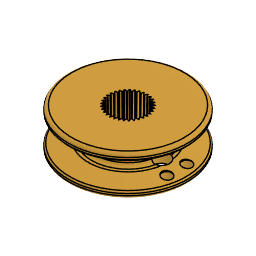
Spool_v5 (Autodesk Fusion 360 design; units mm, degrees)
Autodesk Fusion 360 part; units mm, degrees
note: some values were not read from the file. Set by a fixed rule: which sketch regions a step uses.
sketch "Sketch1" plane through (0, 0, 0) normal (0, 0, 1) x (1, 0, 0)
  line L0 (-0.0246, -2.4999) -> (0.1607, -2.8207)
  line L1 (0.1607, -2.8207) -> (0.3083, -2.4809)
  arc A0 (0.3083, -2.4809) -> (0.449, -2.4594) centre (0, 0) ccw
  line L2 (0.449, -2.4594) -> (0.6916, -2.7393)
  line L3 (0.6916, -2.7393) -> (0.7722, -2.3777)
  arc A1 (0.7722, -2.3777) -> (0.9063, -2.3299) centre (0, 0) ccw
  line L4 (0.9063, -2.3299) -> (1.1975, -2.5589)
  line L5 (1.1975, -2.5589) -> (1.2083, -2.1886)
  arc A2 (1.2083, -2.1886) -> (1.3309, -2.1163) centre (0, 0) ccw
  line L6 (1.3309, -2.1163) -> (1.6601, -2.286)
  line L7 (1.6601, -2.286) -> (1.6006, -1.9204)
  arc A3 (1.6006, -1.9204) -> (1.7073, -1.8262) centre (0, 0) ccw
  line L8 (1.7073, -1.8262) -> (2.0628, -1.9306)
  line L9 (2.0628, -1.9306) -> (1.9351, -1.5828)
  arc A4 (1.9351, -1.5828) -> (2.0221, -1.4701) centre (0, 0) ccw
  line L10 (2.0221, -1.4701) -> (2.3909, -1.5053)
  line L11 (2.3909, -1.5053) -> (2.1997, -1.188)
  arc A5 (2.1997, -1.188) -> (2.2638, -1.0608) centre (0, 0) ccw
  line L12 (2.2638, -1.0608) -> (2.6325, -1.0256)
  line L13 (2.6325, -1.0256) -> (2.3848, -0.7502)
  arc A6 (2.3848, -0.7502) -> (2.4236, -0.6133) centre (0, 0) ccw
  line L14 (2.4236, -0.6133) -> (2.7791, -0.5089)
  line L15 (2.7791, -0.5089) -> (2.4837, -0.2853)
  arc A7 (2.4837, -0.2853) -> (2.4959, -0.1435) centre (0, 0) ccw
  line L16 (2.4959, -0.1435) -> (2.8251, 0.0263)
  line L17 (2.8251, 0.0263) -> (2.4928, 0.1899)
  arc A8 (2.4928, 0.1899) -> (2.4779, 0.3314) centre (0, 0) ccw
  line L18 (2.4779, 0.3314) -> (2.7691, 0.5605)
  line L19 (2.7691, 0.5605) -> (2.4118, 0.6582)
  arc A9 (2.4118, 0.6582) -> (2.3704, 0.7944) centre (0, 0) ccw
  line L20 (2.3704, 0.7944) -> (2.613, 1.0744)
  line L21 (2.613, 1.0744) -> (2.2436, 1.1028)
  arc A10 (2.2436, 1.1028) -> (2.1772, 1.2287) centre (0, 0) ccw
  line L22 (2.1772, 1.2287) -> (2.3625, 1.5495)
  line L23 (2.3625, 1.5495) -> (1.9944, 1.5074)
  arc A11 (1.9944, 1.5074) -> (1.9054, 1.6185) centre (0, 0) ccw
  line L24 (1.9054, 1.6185) -> (2.0265, 1.9686)
  line L25 (2.0265, 1.9686) -> (1.6731, 1.8576)
  arc A12 (1.6731, 1.8576) -> (1.5646, 1.9498) centre (0, 0) ccw
  line L26 (1.5646, 1.9498) -> (1.6173, 2.3165)
  line L27 (1.6173, 2.3165) -> (1.2913, 2.1407)
  arc A13 (1.2913, 2.1407) -> (1.1674, 2.2107) centre (0, 0) ccw
  line L28 (1.1674, 2.2107) -> (1.1497, 2.5807)
  line L29 (1.1497, 2.5807) -> (0.8628, 2.3464)
  arc A14 (0.8628, 2.3464) -> (0.7279, 2.3917) centre (0, 0) ccw
  line L30 (0.7279, 2.3917) -> (0.6405, 2.7517)
  line L31 (0.6405, 2.7517) -> (0.4032, 2.4673)
  arc A15 (0.4032, 2.4673) -> (0.2621, 2.4862) centre (0, 0) ccw
  line L32 (0.2621, 2.4862) -> (0.1082, 2.8232)
  line L33 (0.1082, 2.8232) -> (-0.0711, 2.499)
  arc A16 (-0.0711, 2.499) -> (-0.2132, 2.4909) centre (0, 0) ccw
  line L34 (-0.2132, 2.4909) -> (-0.4281, 2.7926)
  line L35 (-0.4281, 2.7926) -> (-0.5427, 2.4404)
  arc A17 (-0.5427, 2.4404) -> (-0.6807, 2.4055) centre (0, 0) ccw
  line L36 (-0.6807, 2.4055) -> (-0.9488, 2.6612)
  line L37 (-0.9488, 2.6612) -> (-0.9948, 2.2936)
  arc A18 (-0.9948, 2.2936) -> (-1.1237, 2.2332) centre (0, 0) ccw
  line L38 (-1.1237, 2.2332) -> (-1.4353, 2.4335)
  line L39 (-1.4353, 2.4335) -> (-1.4108, 2.0639)
  arc A19 (-1.4108, 2.0639) -> (-1.526, 1.9802) centre (0, 0) ccw
  line L40 (-1.526, 1.9802) -> (-1.8699, 2.1179)
  line L41 (-1.8699, 2.1179) -> (-1.7759, 1.7596)
  arc A20 (-1.7759, 1.7596) -> (-1.8732, 1.6556) centre (0, 0) ccw
  line L42 (-1.8732, 1.6556) -> (-2.2369, 1.7257)
  line L43 (-2.2369, 1.7257) -> (-2.0768, 1.3917)
  arc A21 (-2.0768, 1.3917) -> (-2.1527, 1.2712) centre (0, 0) ccw
  line L44 (-2.1527, 1.2712) -> (-2.5231, 1.2712)
  line L45 (-2.5231, 1.2712) -> (-2.3027, 0.9735)
  arc A22 (-2.3027, 0.9735) -> (-2.3543, 0.8409) centre (0, 0) ccw
  line L46 (-2.3543, 0.8409) -> (-2.7181, 0.7707)
  line L47 (-2.7181, 0.7707) -> (-2.4453, 0.5201)
  arc A23 (-2.4453, 0.5201) -> (-2.4709, 0.3801) centre (0, 0) ccw
  line L48 (-2.4709, 0.3801) -> (-2.8148, 0.2424)
  line L49 (-2.8148, 0.2424) -> (-2.4995, 0.0479)
  arc A24 (-2.4995, 0.0479) -> (-2.4982, -0.0944) centre (0, 0) ccw
  line L50 (-2.4982, -0.0944) -> (-2.8098, -0.2947)
  line L51 (-2.8098, -0.2947) -> (-2.4634, -0.426)
  arc A25 (-2.4634, -0.426) -> (-2.4352, -0.5655) centre (0, 0) ccw
  line L52 (-2.4352, -0.5655) -> (-2.7033, -0.8211)
  line L53 (-2.7033, -0.8211) -> (-2.3383, -0.8845)
  arc A26 (-2.3383, -0.8845) -> (-2.2842, -1.0161) centre (0, 0) ccw
  line L54 (-2.2842, -1.0161) -> (-2.499, -1.3179)
  line L55 (-2.499, -1.3179) -> (-2.1287, -1.311)
  arc A27 (-2.1287, -1.311) -> (-2.0506, -1.4301) centre (0, 0) ccw
  line L56 (-2.0506, -1.4301) -> (-2.2045, -1.767)
  line L57 (-2.2045, -1.767) -> (-1.8421, -1.6902)
  arc A28 (-1.8421, -1.6902) -> (-1.7429, -1.7923) centre (0, 0) ccw
  line L58 (-1.7429, -1.7923) -> (-1.8302, -2.1523)
  line L59 (-1.8302, -2.1523) -> (-1.4889, -2.0083)
  arc A29 (-1.4889, -2.0083) -> (-1.3722, -2.0897) centre (0, 0) ccw
  line L60 (-1.3722, -2.0897) -> (-1.3898, -2.4598)
  line L61 (-1.3898, -2.4598) -> (-1.0819, -2.2538)
  arc A30 (-1.0819, -2.2538) -> (-0.9519, -2.3117) centre (0, 0) ccw
  line L62 (-0.9519, -2.3117) -> (-0.8992, -2.6783)
  line L63 (-0.8992, -2.6783) -> (-0.6359, -2.4178)
  arc A31 (-0.6359, -2.4178) -> (-0.4972, -2.4501) centre (0, 0) ccw
  line L64 (-0.4972, -2.4501) -> (-0.3761, -2.8001)
  line L65 (-0.3761, -2.8001) -> (-0.1668, -2.4944)
  arc A32 (-0.1668, -2.4944) -> (-0.0246, -2.4999) centre (0, 0) ccw
  circle A33 centre (0, 0) radius 9
  circle A34 centre (0, 0) radius 5
  circle A35 centre (5, 0) radius 1.25
  circle A36 centre (0, 0) radius 1.7
  line L66 (7.3721, -1.5) -> (7.3721, 1.5)
  circle A37 centre (7.3721, -1.5) radius 0.75
  circle A38 centre (7.3721, 1.5) radius 0.75
  line L67 (7.3721, -1.5) -> (7.3721, -2.25)
  arc A39 (1.6851, 1.9138) -> (1.6182, 1.9708) centre (0, 0) ccw
  line L68 (1.6182, 1.9708) -> (1.6809, 2.4076)
  line L69 (1.6809, 2.4076) -> (1.2925, 2.1982)
  arc A40 (1.2925, 2.1982) -> (1.2159, 2.2414) centre (0, 0) ccw
  line L70 (1.2159, 2.2414) -> (1.1949, 2.6822)
  line L71 (1.1949, 2.6822) -> (0.8531, 2.4031)
  arc A41 (0.8531, 2.4031) -> (0.7698, 2.431) centre (0, 0) ccw
  line L72 (0.7698, 2.431) -> (0.6657, 2.8599)
  line L73 (0.6657, 2.8599) -> (0.3829, 2.5211)
  arc A42 (0.3829, 2.5211) -> (0.2958, 2.5328) centre (0, 0) ccw
  line L74 (0.2958, 2.5328) -> (0.1124, 2.9342)
  line L75 (0.1124, 2.9342) -> (-0.1011, 2.548)
  arc A43 (-0.1011, 2.548) -> (-0.1889, 2.543) centre (0, 0) ccw
  line L76 (-0.1889, 2.543) -> (-0.4449, 2.9025)
  line L77 (-0.4449, 2.9025) -> (-0.5815, 2.4828)
  arc A44 (-0.5815, 2.4828) -> (-0.6667, 2.4613) centre (0, 0) ccw
  line L78 (-0.6667, 2.4613) -> (-0.9862, 2.7658)
  line L79 (-0.9862, 2.7658) -> (-1.0409, 2.3279)
  arc A45 (-1.0409, 2.3279) -> (-1.1205, 2.2906) centre (0, 0) ccw
  line L80 (-1.1205, 2.2906) -> (-1.4918, 2.5292)
  line L81 (-1.4918, 2.5292) -> (-1.4626, 2.0888)
  arc A46 (-1.4626, 2.0888) -> (-1.5337, 2.0372) centre (0, 0) ccw
  line L82 (-1.5337, 2.0372) -> (-1.9435, 2.2012)
  line L83 (-1.9435, 2.2012) -> (-1.8315, 1.7743)
  arc A47 (-1.8315, 1.7743) -> (-1.8916, 1.7101) centre (0, 0) ccw
  line L84 (-1.8916, 1.7101) -> (-2.3249, 1.7936)
  line L85 (-2.3249, 1.7936) -> (-2.1342, 1.3956)
  arc A48 (-2.1342, 1.3956) -> (-2.181, 1.3212) centre (0, 0) ccw
  line L86 (-2.181, 1.3212) -> (-2.6223, 1.3212)
  line L87 (-2.6223, 1.3212) -> (-2.3597, 0.9665)
  arc A49 (-2.3597, 0.9665) -> (-2.3917, 0.8846) centre (0, 0) ccw
  line L88 (-2.3917, 0.8846) -> (-2.825, 0.801)
  line L89 (-2.825, 0.801) -> (-2.5, 0.5025)
  arc A50 (-2.5, 0.5025) -> (-2.5158, 0.416) centre (0, 0) ccw
  line L90 (-2.5158, 0.416) -> (-2.9255, 0.2519)
  line L91 (-2.9255, 0.2519) -> (-2.5499, 0.0203)
  arc A51 (-2.5499, 0.0203) -> (-2.5491, -0.0677) centre (0, 0) ccw
  line L92 (-2.5491, -0.0677) -> (-2.9204, -0.3063)
  line L93 (-2.9204, -0.3063) -> (-2.5077, -0.4627)
  arc A52 (-2.5077, -0.4627) -> (-2.4902, -0.5489) centre (0, 0) ccw
  line L94 (-2.4902, -0.5489) -> (-2.8096, -0.8534)
  line L95 (-2.8096, -0.8534) -> (-2.3748, -0.9289)
  arc A53 (-2.3748, -0.9289) -> (-2.3414, -1.0102) centre (0, 0) ccw
  line L96 (-2.3414, -1.0102) -> (-2.5973, -1.3697)
  line L97 (-2.5973, -1.3697) -> (-2.1561, -1.3616)
  arc A54 (-2.1561, -1.3616) -> (-2.1079, -1.4351) centre (0, 0) ccw
  line L98 (-2.1079, -1.4351) -> (-2.2912, -1.8365)
  line L99 (-2.2912, -1.8365) -> (-1.8594, -1.745)
  arc A55 (-1.8594, -1.745) -> (-1.7982, -1.8081) centre (0, 0) ccw
  line L100 (-1.7982, -1.8081) -> (-1.9022, -2.2369)
  line L101 (-1.9022, -2.2369) -> (-1.4956, -2.0654)
  arc A56 (-1.4956, -2.0654) -> (-1.4235, -2.1157) centre (0, 0) ccw
  line L102 (-1.4235, -2.1157) -> (-1.4445, -2.5565)
  line L103 (-1.4445, -2.5565) -> (-1.0777, -2.3111)
  arc A57 (-1.0777, -2.3111) -> (-0.9974, -2.3469) centre (0, 0) ccw
  line L104 (-0.9974, -2.3469) -> (-0.9345, -2.7837)
  line L105 (-0.9345, -2.7837) -> (-0.6208, -2.4733)
  arc A58 (-0.6208, -2.4733) -> (-0.5352, -2.4932) centre (0, 0) ccw
  line L106 (-0.5352, -2.4932) -> (-0.3908, -2.9102)
  line L107 (-0.3908, -2.9102) -> (-0.1416, -2.5461)
  arc A59 (-0.1416, -2.5461) -> (-0.0537, -2.5494) centre (0, 0) ccw
  line L108 (-0.0537, -2.5494) -> (0.167, -2.9316)
  line L109 (0.167, -2.9316) -> (0.3428, -2.5268)
  arc A60 (0.3428, -2.5268) -> (0.4298, -2.5135) centre (0, 0) ccw
  line L110 (0.4298, -2.5135) -> (0.7188, -2.847)
  line L111 (0.7188, -2.847) -> (0.8149, -2.4163)
  arc A61 (0.8149, -2.4163) -> (0.8977, -2.3868) centre (0, 0) ccw
  line L112 (0.8977, -2.3868) -> (1.2446, -2.6596)
  line L113 (1.2446, -2.6596) -> (1.2574, -2.2184)
  arc A62 (1.2574, -2.2184) -> (1.3332, -2.1738) centre (0, 0) ccw
  line L114 (1.3332, -2.1738) -> (1.7254, -2.376)
  line L115 (1.7254, -2.376) -> (1.6545, -1.9404)
  arc A63 (1.6545, -1.9404) -> (1.7204, -1.8822) centre (0, 0) ccw
  line L116 (1.7204, -1.8822) -> (2.1439, -2.0065)
  line L117 (2.1439, -2.0065) -> (1.9919, -1.5922)
  arc A64 (1.9919, -1.5922) -> (2.0456, -1.5226) centre (0, 0) ccw
  line L118 (2.0456, -1.5226) -> (2.4849, -1.5645)
  line L119 (2.4849, -1.5645) -> (2.2572, -1.1864)
  arc A65 (2.2572, -1.1864) -> (2.2967, -1.1079) centre (0, 0) ccw
  line L120 (2.2967, -1.1079) -> (2.7361, -1.0659)
  line L121 (2.7361, -1.0659) -> (2.4409, -0.7378)
  arc A66 (2.4409, -0.7378) -> (2.4649, -0.6532) centre (0, 0) ccw
  line L122 (2.4649, -0.6532) -> (2.8883, -0.5289)
  line L123 (2.8883, -0.5289) -> (2.5364, -0.2625)
  arc A67 (2.5364, -0.2625) -> (2.544, -0.1749) centre (0, 0) ccw
  line L124 (2.544, -0.1749) -> (2.9362, 0.0273)
  line L125 (2.9362, 0.0273) -> (2.5403, 0.2222)
  arc A68 (2.5403, 0.2222) -> (2.5311, 0.3097) centre (0, 0) ccw
  line L126 (2.5311, 0.3097) -> (2.878, 0.5825)
  line L127 (2.878, 0.5825) -> (2.4523, 0.699)
  arc A69 (2.4523, 0.699) -> (2.4268, 0.7831) centre (0, 0) ccw
  line L128 (2.4268, 0.7831) -> (2.7158, 1.1166)
  line L129 (2.7158, 1.1166) -> (2.2757, 1.1504)
  arc A70 (2.2757, 1.1504) -> (2.2347, 1.2282) centre (0, 0) ccw
  line L130 (2.2347, 1.2282) -> (2.4554, 1.6104)
  line L131 (2.4554, 1.6104) -> (2.0169, 1.5603)
  arc A71 (2.0169, 1.5603) -> (1.9619, 1.6289) centre (0, 0) ccw
  line L132 (1.9619, 1.6289) -> (2.1062, 2.046)
  line L133 (2.1062, 2.046) -> (1.6851, 1.9138)
  point P0 (7.3721, 0)
  dimension "d1" = 0.05
  dimension "d2" = 18
  dimension "d5" = 10
  dimension "d10" = 2.5
  dimension "d19" = 3.4
  dimension "d24" = 3
  dimension "d25" = 1.5
  dimension "d26" = 1.5
  constraint concentric A0 A33
  constraint concentric A0 A34
  constraint coincident A34 A35.centre
  constraint concentric A33 A36
  constraint midpoint L66 P0
  constraint vertical L66
  constraint coincident L66.start A37.centre
  constraint coincident L66.end A38.centre
  constraint coincident A37 L67.end
  constraint parallel L66 L67
  measures "d2" diameter of A33
  measures "d5" diameter of A34
  measures "d10" diameter of A35
  measures "d19" diameter of A36
  measures "d24" distance of L66.start L66.end
  measures "d25" diameter of A37
  measures "d26" diameter of A38
extrude "Extrude1" add sketch "Sketch1" along normal blind 6 contours A33 | A34 A35 | A34 A35 | A34 A35 | L66 A37 L67 | L66 A37 L67 | A38
extrude "Extrude2" cut sketch "Sketch1" along normal blind 3 from surface at 1.5 contours A33 | A34 A35 | L66 A37 L67 | L66 A37 L67 | A38 picked at (5.374, -0.3105)
extrude "Extrude3" cut sketch "Sketch1" along normal blind 4.5 contours L0 L1 A0 L2 L3 A1 L4 L5 A2 L6 L7 A3 L8 L9 A4 L10 L11 A5 L12 L13 A6 L14 L15 A7 L16 L17 A8 L18 L19 A9 L20 L21 A10 L22 L23 A11 L24 L25 A12 L26 L27 A13 L28 L29 A14 L30 L31 A15 L32 L33 A16 L34 L35 A17 L36 L37 A18 L38 L39 A19 L40 L41 A20 L42 L43 A21 L44 L45 A22 L46 L47 A23 L48 L49 A24 L50 L51 A25 L52 L53 A26 L54 L55 A27 L56 L57 A28 L58 L59 A29 L60 L61 A30 L62 L63 A31 L64 L65 A32 | A34 A35 | A34 A35 | A36 | L66 A37 L67 | L66 A37 L67 | A38 | A39 L68 L69 A40 L70 L71 A41 L72 L73 A42 L74 L75 A43 L76 L77 A44 L78 L79 A45 L80 L81 A46 L82 L83 A47 L84 L85 A48 L86 L87 A49 L88 L89 A50 L90 L91 A51 L92 L93 A52 L94 L95 A53 L96 L97 A54 L98 L99 A55 L100 L101 A56 L102 L103 A57 L104 L105 A58 L106 L107 A59 L108 L109 A60 L110 L111 A61 L112 L113 A62 L114 L115 A63 L116 L117 A64 L118 L119 A65 L120 L121 A66 L122 L123 A67 L124 L125 A68 L126 L127 A69 L128 L129 A70 L130 L131 A71 L132 L133 picked at (4.5948, -0.2579) picked at (5.374, -0.3105)
fillet "Fillet2" radius 0.5 2 edges at (-8.3909, -3.2545, 0) (-8.3909, -3.2545, 6)
chamfer "Chamfer1" distance 0.5 distance2 3 2 edges at (-8.3909, 3.2545, 1.5) (-8.3909, -3.2545, 4.5) measured on face at (8.9553, -0.8961, 0.8333) measured on face at (8.9553, -0.8961, 4.8333) tangent chain off
fillet "Fillet4" radius 0.5 2 edges at (-5, 0, 1.5) (-5, 0, 4.5)
extrude "Extrude4" add sketch "Sketch1" along normal blind 2 contours L0 L1 A0 L2 L3 A1 L4 L5 A2 L6 L7 A3 L8 L9 A4 L10 L11 A5 L12 L13 A6 L14 L15 A7 L16 L17 A8 L18 L19 A9 L20 L21 A10 L22 L23 A11 L24 L25 A12 L26 L27 A13 L28 L29 A14 L30 L31 A15 L32 L33 A16 L34 L35 A17 L36 L37 A18 L38 L39 A19 L40 L41 A20 L42 L43 A21 L44 L45 A22 L46 L47 A23 L48 L49 A24 L50 L51 A25 L52 L53 A26 L54 L55 A27 L56 L57 A28 L58 L59 A29 L60 L61 A30 L62 L63 A31 L64 L65 A32 | A39 L68 L69 A40 L70 L71 A41 L72 L73 A42 L74 L75 A43 L76 L77 A44 L78 L79 A45 L80 L81 A46 L82 L83 A47 L84 L85 A48 L86 L87 A49 L88 L89 A50 L90 L91 A51 L92 L93 A52 L94 L95 A53 L96 L97 A54 L98 L99 A55 L100 L101 A56 L102 L103 A57 L104 L105 A58 L106 L107 A59 L108 L109 A60 L110 L111 A61 L112 L113 A62 L114 L115 A63 L116 L117 A64 L118 L119 A65 L120 L121 A66 L122 L123 A67 L124 L125 A68 L126 L127 A69 L128 L129 A70 L130 L131 A71 L132 L133
fillet "Fillet3" radius 0.5 1 edges at (-1.585, 0.6147, 2)
fillet "Fillet5" radius 0.25 2 edges at (-8.3909, -3.2545, 1) (-8.3909, 3.2545, 5)
chamfer "Chamfer2" distance 0.05 distance2 4 33 edges at (-1.8618, 1.7425, 6) (-1.4984, 2.0633, 6) (-1.0808, 2.3096, 6) (-0.6242, 2.4724, 6) (-0.145, 2.5459, 6) (0.3394, 2.5273, 6) (0.8116, 2.4174, 6) (1.2544, 2.2201, 6) (1.6519, 1.9426, 6) (1.9897, 1.5949, 6) (2.2556, 1.1895, 6) (2.4399, 0.7411, 6) (2.5361, 0.266, 6) (2.5406, -0.2188, 6) (2.4533, -0.6956, 6) (2.2773, -1.1474, 6) (2.019, -1.5576, 6) (1.6877, -1.9116, 6) (1.2955, -2.1964, 6) (0.8564, -2.4019, 6) (0.3864, -2.5206, 6) (-0.0976, -2.5481, 6) (-0.5781, -2.4836, 6) (-1.0377, -2.3293, 6) (-1.4598, -2.0908, 6) (-1.8291, -1.7768, 6) (-2.1323, -1.3985, 6) (-2.3584, -0.9697, 6) (-2.4993, -0.5059, 6) (-2.5499, -0.0237, 6) (-2.5083, 0.4593, 6) (-2.376, 0.9257, 6) (-2.1579, 1.3586, 6) measured on face at (-5.1817, -4.1354, 6) measured on face at (-5.1817, -4.1354, 6) measured on face at (-5.1817, -4.1354, 6) measured on face at (-5.1817, -4.1354, 6) measured on face at (-5.1817, -4.1354, 6) measured on face at (-5.1817, -4.1354, 6) measured on face at (-5.1817, -4.1354, 6) measured on face at (-5.1817, -4.1354, 6) measured on face at (-5.1817, -4.1354, 6) measured on face at (-5.1817, -4.1354, 6) measured on face at (-5.1817, -4.1354, 6) measured on face at (-5.1817, -4.1354, 6) measured on face at (-5.1817, -4.1354, 6) measured on face at (-5.1817, -4.1354, 6) measured on face at (-5.1817, -4.1354, 6) measured on face at (-5.1817, -4.1354, 6) measured on face at (-5.1817, -4.1354, 6) measured on face at (-5.1817, -4.1354, 6) measured on face at (-5.1817, -4.1354, 6) measured on face at (-5.1817, -4.1354, 6) measured on face at (-5.1817, -4.1354, 6) measured on face at (-5.1817, -4.1354, 6) measured on face at (-5.1817, -4.1354, 6) measured on face at (-5.1817, -4.1354, 6) measured on face at (-5.1817, -4.1354, 6) measured on face at (-5.1817, -4.1354, 6) measured on face at (-5.1817, -4.1354, 6) measured on face at (-5.1817, -4.1354, 6) measured on face at (-5.1817, -4.1354, 6) measured on face at (-5.1817, -4.1354, 6) measured on face at (-5.1817, -4.1354, 6) measured on face at (-5.1817, -4.1354, 6) measured on face at (-5.1817, -4.1354, 6) tangent chain off
chamfer "Chamfer3" distance 0.1 distance2 1.2 2 edges at (6.6729, 1.2288, 0) (6.6729, -1.7712, 0) measured on face at (3.5782, -3.0191, 0) measured on face at (3.5782, -3.0191, 0) tangent chain off
